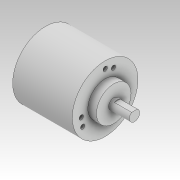
# Autodesk Inventor part: TestEncoder
Saved by Autodesk Inventor 2020 (Build 240168000, 168)
## iProperties
Created: 2022-01-16
Part Number: TestEncoder
Material: Generic
Document SubType Name: Modeling
Designer: DDeGo
Density: 1 g/cm^3
Appearance: Default
Author: DDeGo
Autodesk Inventor part; units mm, degrees
ref_plane "YZ Plane" through (0, 0, 0) normal (1, 0, 0) x (0, 1, 0)
ref_plane "XZ Plane" through (0, 0, 0) normal (0, 1, 0) x (-1, 0, 0)
ref_plane "XY Plane" through (0, 0, 0) normal (0, 0, 1) x (1, 0, 0)
sketch "Sketch1" plane through (0, 0, 0) normal (0, 0, 1) x (1, 0, 0)
  line L0 (0, 0) -> (0, 19)
  line L1 (0, 19) -> (34.5, 19)
  line L2 (34.5, 19) -> (34.5, 10)
  line L3 (34.5, 10) -> (39.5, 10)
  line L4 (39.5, 10) -> (39.5, 3)
  line L5 (39.5, 3) -> (51.5, 3)
  line L6 (51.5, 3) -> (51.5, 0)
  line L7 (51.5, 0) -> (0, 0)
  dimension "d0" = 19
  dimension "d1" = 34.5
  dimension "d2" = 5
  dimension "d3" = 10
  dimension "d4" = 12
  dimension "d5" = 3
  constraints: 16 end point, 7 perpendicular, 1 vertical
  measures "d0" distance between parallel lines of L7 L1
  measures "d1" distance between parallel lines of L0 L2
  measures "d2" distance of L2.end L3.end
  measures "d3" distance between parallel lines of L3 L7
  measures "d4" distance of L4.end L5.end
  measures "d5" distance between parallel lines of L7 L5
revolve "Revolution1" add sketch "Sketch1" angle 360 about axis through (51.5, 0, 0) along (-1, 0, 0)
sketch "Sketch2" plane through (51.5, 0, 0) normal (1, 0, 0) x (0, 0, -1)
  circle A0 centre (0, 0) radius 3 projected
  circle A1 centre (0, 0) radius 3 projected
  line L0 (-1.6583, 2.5) -> (1.6583, 2.5)
  point P0 (0, 0)
  point P1 (-1.6583, 2.5)
  point P2 (1.6583, 2.5)
  dimension "d7" = 2.5
  constraints: 2 end point, 2 point on circle, 1 horizontal
  measures "d7" distance from line of L0 point (0, 0)
extrude "Extrusion1" cut sketch "Sketch2" against normal blind 10 contours L0 A0 picked at (-0.1169, 2.6598)
sketch "Sketch3" plane through (34.5, 0, 0) normal (1, 0, 0) x (0, 0, -1)
  circle A0 centre (0, 15) radius 1.25
  circle A1 centre (4.7883, 13.1557) radius 1.25
  circle A2 centre (0, 0) radius 3 projected
  circle A3 centre (0, 0) radius 14 construction
  circle A4 centre (0, 0) radius 15 construction
  circle A5 centre (0, 0) radius 19 projected
  line L0 (0, 0) -> (0, 15) construction
  line L1 (1.6583, 2.5) -> (-1.6583, 2.5) projected
  line L2 (0, 0) -> (4.7883, 13.1557) construction
  circle A6 centre (-13.7873, -2.4311) radius 1.25
  circle A7 centre (-12.9904, -7.5) radius 1.25
  circle A8 centre (8.999, -10.7246) radius 1.25
  circle A9 centre (12.9904, -7.5) radius 1.25
  dimension "d21" = 28
  dimension "d22" = 30
  dimension "d10" = 4
  dimension "d11" = 5
  dimension "d12" = 2.5
  dimension "d13" = 2.5
  dimension "d14" = 20
  dimension "d17" = 360
  constraints: 6 centre point, 4 end point, 2 coincident, 1 perpendicular, 1 vertical alignment, 18 other
  measures "d12" diameter of A0
  measures "d13" diameter of A1
  measures "d14" angle of L2 L0
extrude "Extrusion2" cut sketch "Sketch3" against normal blind 10 contours A0 | A1 | A2 L1 | L1 A2 | A6 | A7 | A8 | A9
body "Solid1"
